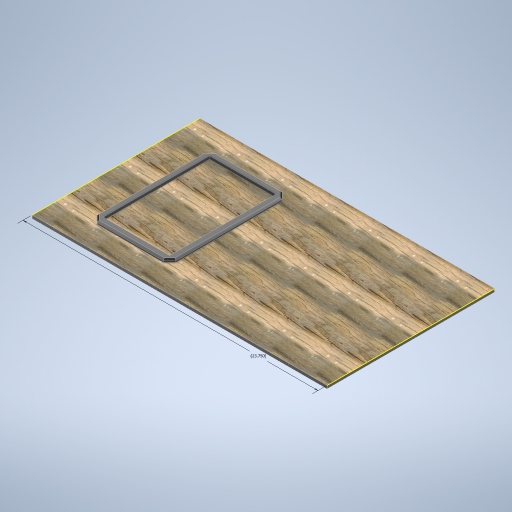
# Autodesk Inventor part: UpperHalfofFrontBack_Ocampo
Saved by Autodesk Inventor 2023 (Build 270158000, 158)
## iProperties
Created: 2025-03-05
Part Number: UpperHalfofFrontBack_Ocampo
Material: Generic
Document SubType Name: Modeling
Designer: FrameUser
Density: 1 g/cm^3
Appearance: Fine Textured - Black
Author: FrameUser
Autodesk Inventor part; units mm, degrees
ref_plane "YZ Plane" through (0, 0, 0) normal (1, 0, 0) x (0, 1, 0)
ref_plane "XZ Plane" through (0, 0, 0) normal (0, 1, 0) x (-1, 0, 0)
ref_plane "XY Plane" through (0, 0, 0) normal (0, 0, 1) x (1, 0, 0)
sketch "Sketch1" plane through (0, 0, 0) normal (0, 1, 0) x (-1, 0, 0)
  line L0 (0, 0) -> (-609.6, 0)
  line L1 (-609.6, 0) -> (-609.6, -342.9)
  line L2 (-609.6, -342.9) -> (0, -342.9)
  line L3 (0, -342.9) -> (0, 0)
  dimension "d0" = 609.6
  dimension "d1" = 342.9
  dimension "d2" = 609.6
  constraints: 8 end point, 2 horizontal, 1 vertical
  measures "d0" distance of L0.start L0.end
  measures "d1" distance of L0.end L1.end
  measures "d2" distance of L1.end L2.end
extrude "Extrusion1" add sketch "Sketch1" along normal blind 6.35
sketch "Sketch2" plane through (0, 0, 0) normal (0, 1, 0) x (-1, 0, 0)
  line L0 (-609.6, -342.9) -> (0, -342.9) projected
  line L1 (0, 0) -> (-609.6, 0) projected
  line L2 (-609.6, -342.9) -> (-603.25, -342.9)
  line L3 (-603.25, -342.9) -> (-603.25, 0)
  line L4 (-603.25, 0) -> (-609.6, 0)
  line L5 (-609.6, 0) -> (-609.6, -342.9)
  dimension "d5" = 6.35
  constraints: 8 end point, 2 parallel, 1 horizontal, 1 perpendicular, 1 point on line
  measures "d5" distance of L4.end L3.end
extrude "Extrusion2" cut sketch "Sketch2" along normal blind 231.775
sketch "Sketch3" plane through (0, 6.35, 0) normal (0, 1, 0) x (1, 0, 0)
  line L0 (603.25, 0) -> (603.25, 342.9) projected
  line L1 (0, 342.9) -> (0, 0) projected
  dimension "d8" = 603.25
  measures "d8" distance between parallel lines of L0 L1
sketch "Sketch4" plane through (0, 6.35, 0) normal (0, 1, 0) x (1, 0, 0)
  line L0 (603.25, 342.9) -> (0, 342.9) projected
  line L1 (0, 0) -> (603.25, 0) projected
  line L2 (0, 342.9) -> (0, 0) projected
  line L3 (0, 0) -> (301.625, 0)
  line L4 (301.625, 0) -> (301.625, 342.9)
  line L5 (301.625, 0) -> (452.4375, 0)
  line L6 (82.8675, 171.45) -> (82.8675, 280.162)
  line L7 (82.8675, 280.162) -> (150.8125, 280.162)
  line L8 (82.8675, 171.45) -> (82.8675, 62.738)
  line L9 (82.8675, 62.738) -> (150.8125, 62.738)
  line L10 (218.7575, 280.162) -> (150.8125, 280.162)
  line L11 (218.7575, 171.45) -> (218.7575, 280.162)
  line L12 (218.7575, 171.45) -> (218.7575, 62.738)
  line L13 (218.7575, 62.738) -> (150.8125, 62.738)
  line L14 (218.7575, 280.162) -> (218.7575, 292.862)
  line L15 (218.7575, 292.862) -> (82.8675, 292.862)
  line L16 (82.8675, 292.862) -> (82.8675, 280.162)
  line L17 (87.7385, 280.162) -> (75.0385, 280.162)
  line L18 (77.9965, 62.738) -> (87.7385, 62.738)
  line L19 (82.8675, 280.162) -> (70.1675, 280.162)
  line L20 (70.1675, 280.162) -> (70.1675, 62.738)
  line L21 (70.1675, 62.738) -> (82.8675, 62.738)
  line L22 (82.8675, 62.738) -> (82.8675, 50.038)
  line L23 (82.8675, 50.038) -> (218.7575, 50.038)
  line L24 (218.7575, 50.038) -> (218.7575, 62.738)
  line L25 (218.7575, 62.738) -> (231.4575, 62.738)
  line L26 (231.4575, 62.738) -> (231.4575, 280.162)
  line L27 (231.4575, 280.162) -> (218.7575, 280.162)
  line L28 (231.4575, 62.738) -> (218.7575, 50.038)
  line L29 (82.8675, 50.038) -> (70.1675, 62.738)
  line L30 (70.1675, 62.738) -> (70.1675, 280.162)
  line L31 (82.8675, 292.862) -> (70.1675, 280.162)
  line L32 (218.7575, 292.862) -> (231.4575, 280.162)
  dimension "d9" = 342.9
  dimension "d10" = 301.625
  dimension "d11" = 150.8125
  constraints: 60 end point, 8 point on line, 2 midpoint
  measures "d9" distance between parallel lines of L0 L1
  measures "d10" distance of L1.start L3.end
  measures "d11" distance of L3.end L5.end
extrude "Extrusion3" add sketch "Sketch4" along normal blind 6.35 contours L8 L18 L21 L20 L19 L17 L6 | L16 L15 L14 L10 L7 | L17 L19 L31 L16 | L22 L29 L21 L18 | L9 L13 L24 L23 L22 | L32 L27 L14 | L24 L25 L28 | L27 L26 L25 L12 L11
chamfer "Chamfer1" distance 3.175 angle 45 8 edges at (70.1675, 12.7, -171.45) (76.5175, 12.7, -286.512) (150.8125, 12.7, -292.862) (225.1075, 12.7, -286.512) (231.4575, 12.7, -171.45) (225.1075, 12.7, -56.388) (150.8125, 12.7, -50.038) (76.5175, 12.7, -56.388)
body "Solid1"
